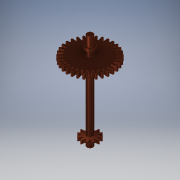
# Autodesk Inventor part: GearConnector
Saved by Autodesk Inventor 2018.1 (Build 221171000, 171)
## iProperties
Created: 2017-09-02
Part Number: GearConnector
Material: Generic
Document SubType Name: Modeling
Designer: ToreDenStore
Density: 1 g/cm^3
Appearance: Default
Author: ToreDenStore
Autodesk Inventor part; units mm, degrees
ref_plane "YZ Plane" through (0, 0, 0) normal (1, 0, 0) x (0, 1, 0)
ref_plane "XZ Plane" through (0, 0, 0) normal (0, 1, 0) x (-1, 0, 0)
ref_plane "XY Plane" through (0, 0, 0) normal (0, 0, 1) x (1, 0, 0)
sketch "Sketch1" plane through (0, 0, 0) normal (0, 1, 0) x (-1, 0, 0)
  circle A0 centre (0, 0) radius 16
  line L0 (0, 0) -> (1.1, -15.9621) construction
  line L1 (0, 0) -> (-1.1, -15.9621) construction
  arc A1 (-0.7967, -19.273) -> (0.7967, -19.273) centre (0, -19.2) ccw
  line L2 (-0.7967, -19.273) -> (-1.1, -15.9621)
  line L3 (1.1, -15.9621) -> (0.7967, -19.273)
  line L4 (0, 0) -> (0, -19.2) construction
  line L5 (0, -27.2) -> (0, 23.2) projected
  dimension "d1" = 2.2
  dimension "d2" = 4
  dimension "d3" = 0.8
  dimension "d4" = 32
  constraints: 10 end point, 4 point on circle, 2 centre point, 2 tangent, 1 coincident, 1 collinear, 1 equal length
  measures "d1" distance of L1.end L0.end
  measures "d3" radius of A1
  measures "d4" diameter of A0
extrude "Extrusion1" add sketch "Sketch1" along normal blind 4
pattern_circular "Circular Pattern1" count 32 over 360 about axis through (0, 0, 0) along (0, 1, 0) of "Extrusion1"
sketch "Sketch2" plane through (0, 4, 0) normal (0, 1, 0) x (1, 0, 0)
  circle A0 centre (0, 0) radius 2.5
  dimension "d10" = 5
  constraints: 1 centre point, 1 coincident
  measures "d10" diameter of A0
extrude "Extrusion2" add sketch "Sketch2" along normal blind 15
ref_plane "Work Plane1" through (0, 11, 0) normal (0, 1, 0) x (1, 0, 0)
sketch "Sketch3" plane through (0, 11, 0) normal (0, 1, 0) x (1, 0, 0)
  circle A0 centre (0, 0) radius 2.5 projected
  circle A1 centre (0, 0) radius 4
  dimension "d14" = 8
  constraints: 1 centre point, 1 coincident
  measures "d14" diameter of A1
extrude "Extrusion3" add sketch "Sketch3" against normal blind 2
sketch "Sketch4" plane through (0, 0, 0) normal (0, -1, 0) x (1, 0, 0)
  circle A0 centre (0, 0) radius 2.5
  dimension "d17" = 5
  constraints: 1 centre point, 1 coincident
  measures "d17" diameter of A0
extrude "Extrusion4" add sketch "Sketch4" along normal blind 62
ref_plane "Work Plane3" through (0, -57, 0) normal (0, -1, 0) x (1, 0, 0)
sketch "Sketch5" plane through (0, -57, 0) normal (0, -1, 0) x (1, 0, 0)
  circle A0 centre (0, 0) radius 2.5 projected
  arc A1 (-0.0228, -4.9999) -> (0.6526, -4.9572) centre (0, 0) ccw construction
  line L0 (0, 0) -> (0.6526, -4.9572) construction
  line L1 (0, 0) -> (-0.6526, -4.9572) construction
  arc A2 (-0.6526, -4.9572) -> (-0.0228, -4.9999) centre (0, 0) ccw construction
  arc A3 (0.6526, -4.9572) -> (-0.6526, -4.9572) centre (0, 0) ccw
  line L2 (-0.6526, -4.9572) -> (-0.3979, -7.4572)
  line L3 (0.6526, -4.9572) -> (0.3979, -7.4572)
  arc A4 (-0.3979, -7.4572) -> (0.3979, -7.4572) centre (0, -7.4167) ccw
  line L4 (0, -28) -> (0, 28) projected
  dimension "d22" = 15
  dimension "d27" = 5
  dimension "d37" = 2.5
  dimension "d38" = 0.4
  dimension "d39" = 0.6299
  dimension "d40" = 7.5
  constraints: 8 end point, 8 point on circle, 4 centre point, 2 tangent, 1 coincident, 1 equal length, 1 other
  measures "d22" angle of L0 L1
  measures "d27" radius of A3
  measures "d37" vertical distance of L0.end L3.end
  measures "d38" radius of A4
  measures "d39" horizontal distance of L1.end A1.start
  measures "d40" angle to the sketch y axis of L1
extrude "Extrusion6" add sketch "Sketch5" against normal blind 3 contours A0 L4 A3 L3 A4 | A0 L4 A4 L2 A3
pattern_circular "Circular Pattern2" count 12 over 360 about axis through (0, 0, 0) along (0, -1, 0) of "Extrusion6"
equation "\"d40\" = 0.5 * d22"
body "Solid1"
